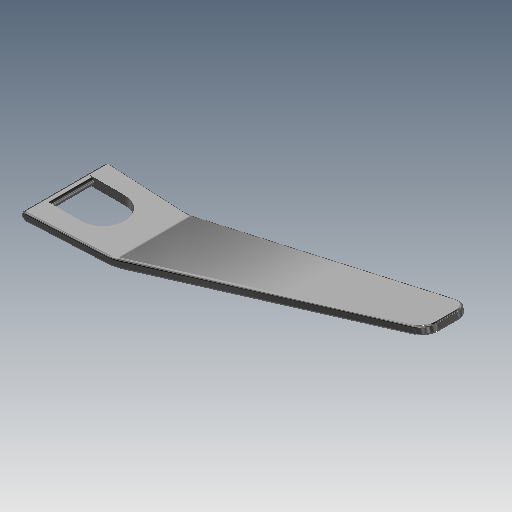
# Autodesk Inventor part: Lever
Saved by Autodesk Inventor 2020.1 (Build 241239000, 239)
## iProperties
Created: 2010-10-13
Part Number: Lever
Document SubType Name: Modeling
Designer: Thom Tremblay
Density: 1 g/cm^3
Material: Generic
Appearance: Chrome - Polished Black
Author: Thom Tremblay
Autodesk Inventor part; units mm, degrees
ref_plane "YZ Plane" through (0, 0, 0) normal (1, 0, 0) x (0, 1, 0)
ref_plane "XZ Plane" through (0, 0, 0) normal (0, 1, 0) x (-1, 0, 0)
ref_plane "XY Plane" through (0, 0, 0) normal (0, 0, 1) x (1, 0, 0)
sketch "Sketch1" plane through (0, 0, 0) normal (0, 0, 1) x (1, 0, 0)
  line L0 (0, 0) -> (5.08, 0)
  line L1 (5.08, 0) -> (22.2542, 4.6018)
  line L2 (5.08, 0) -> (22.86, 0) construction
  line L3 (0, 0) -> (0, 0.508)
  line L4 (0, 0.508) -> (5.0131, 0.508)
  line L5 (5.0131, 0.508) -> (22.1227, 5.0925)
  line L6 (22.1227, 5.0925) -> (22.2542, 4.6018)
  dimension "d0" = 5.08
  dimension "d1" = 17.78
  dimension "d2" = 15
  dimension "d3" = 0.508
  constraints: 14 end point, 3 perpendicular, 2 equal length, 2 horizontal, 1 parallel
  measures "d0" distance of L0.start L0.end
  measures "d1" distance of L0.end L1.end
  measures "d2" angle of L2 L1
  measures "d3" distance of L0.start L3.end
extrude "Extrusion1" add sketch "Sketch1" along normal mid plane 2.54
draft "FaceDraft1" angle 3 pull direction (0.9659258, 0.258819, 0) faces at (10.7824, 1.7033, 1.27) (10.7824, 1.7033, -1.27) fixed edges at (22.1884, 4.8471, 1.27) (22.1884, 4.8471, -1.27)
fillet "Fillet1" radius 3.81 1 edges at (5.08, 0, 0)
fillet "Fillet1" radius 2.54 1 edges at (5.0131, 0.508, 0)
fillet "Fillet1" radius 0.762 2 edges at (22.1884, 4.8471, -1.27) (22.1884, 4.8471, 1.27)
sketch "Sketch2" plane through (4.6787, 0.508, 2.2152) normal (0, 1, 0) x (1, 0, 0)
  line L0 (-4.1707, 3.4852) -> (-2.3927, 3.4852)
  line L1 (-2.3927, 3.4852) -> (-2.3927, 0.9452)
  line L2 (-2.3927, 0.9452) -> (-4.1707, 0.9452)
  line L3 (-4.1707, 0.9452) -> (-4.1707, 3.4852)
  circle A0 centre (-2.3927, 2.2152) radius 1.27
  point P0 (-4.6787, 2.2152)
  dimension "d10" = 2.54
  dimension "d9" = 0.508
  dimension "d11" = 1.778
  constraints: 8 end point, 2 parallel, 1 horizontal, 1 horizontal alignment, 1 midpoint, 1 perpendicular, 1 vertical alignment, 2 other
  measures "d9" distance from line of point (-4.679, 2.215) L3
  measures "d11" distance of L0.start L0.end
extrude "Extrusion2" cut sketch "Sketch2" against normal through all
fillet "Fillet3" radius 0.254 4 edges at (0, 0, 0) (0, 0.508, 0) (0.508, 0.508, 0) (0.508, 0, 0)
fillet "Fillet4" radius 0.127 24 edges at (13.3806, 2.7501, -1.7443) (5.0103, 0.5297, -2.1982) (2.4663, 0.508, -2.3272) (0.0744, 0.4336, -2.4493) (0, 0.254, -2.4555) (0.0744, 0.0744, -2.4542) (2.4162, 0, -2.3367) (5.0757, 0.0326, -2.2016) (13.5606, 2.2724, -1.7417) (22.052, 4.5476, -1.0714) (22.2542, 4.6018, 0) (22.052, 4.5476, 1.0714) (13.5606, 2.2724, 1.7417) (5.0757, 0.0326, 2.2016) (2.4162, 0, 2.3367) (0.0744, 0.4336, 2.4493) (0, 0.254, 2.4555) (0.0744, 0.0744, 2.4542) (2.4663, 0.508, 2.3272) (5.0103, 0.5297, 2.1982) (13.3806, 2.7501, 1.7443) (21.9205, 5.0383, 1.0714) (22.1227, 5.0925, 0) (21.9205, 5.0383, -1.0714)
body "Solid1"
